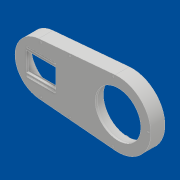
# Autodesk Inventor part: 101-bottom
Saved by Autodesk Inventor 2018 (Build 220112000, 112)
## iProperties
Created: 2019-11-07
Part Number: 101-bottom
Material: Generic
Document SubType Name: Modeling
Designer: Bunny320
Density: 1 g/cm^3
Appearance: Default
Author: Bunny320
Autodesk Inventor part; units mm, degrees
ref_plane "YZ Plane" through (0, 0, 0) normal (1, 0, 0) x (0, 1, 0)
ref_plane "XZ Plane" through (0, 0, 0) normal (0, 1, 0) x (-1, 0, 0)
ref_plane "XY Plane" through (0, 0, 0) normal (0, 0, 1) x (1, 0, 0)
sketch "Sketch2" plane through (0, 0, 0) normal (0, 1, 0) x (-1, 0, 0)
  circle A0 centre (0, 0) radius 45
  circle A1 centre (-141.8, 0) radius 57.5
  line L0 (3.9669, -44.8248) -> (-136.7312, -57.2762)
  line L1 (3.9669, 44.8248) -> (-136.7312, 57.2762)
  dimension "d5" = 141.8
  dimension "d6" = 90
  dimension "d7" = 115
  constraints: 4 end point, 4 point on circle, 4 tangent, 2 centre point, 1 coincident, 1 horizontal alignment
  measures "d5" distance of A1.centre point (0, 0)
  measures "d6" diameter of A0
  measures "d7" diameter of A1
extrude "Extrusion2" add sketch "Sketch2" along normal blind 4
sketch "Sketch5" plane through (0, 4, 0) normal (0, 1, 0) x (1, 0, 0)
  arc A0 (136.7312, -57.2762) -> (136.7312, 57.2762) centre (141.8, 0) ccw projected
  circle A1 centre (141.8, 0) radius 45
  circle A2 centre (141.8, 0) radius 48
  point P0 (0, 0)
  dimension "d17" = 90
  dimension "d18" = 96
  constraints: 2 centre point, 2 coincident
  measures "d17" diameter of A1
  measures "d18" diameter of A2
extrude "Extrusion5" add sketch "Sketch5" along normal blind 14
sketch "Sketch6" plane through (141.8, 4, 0) normal (0, 1, 0) x (1, 0, 0)
  arc A0 (-5.0688, -57.2762) -> (-5.0688, 57.2762) centre (0, 0) ccw projected
  circle A1 centre (0, 0) radius 42
  point P0 (-141.8, 0)
  dimension "d21" = 84
  constraints: 1 centre point, 1 coincident
  measures "d21" diameter of A1
extrude "Extrusion6" cut sketch "Sketch6" against normal through all
sketch "Sketch14" plane through (0, 0, 0) normal (0, 1, 0) x (-1, 0, 0)
  arc A0 (3.9669, -44.8248) -> (3.9669, 44.8248) centre (0, 0) ccw projected
  arc A1 (4.2313, -47.8131) -> (4.2313, 47.8131) centre (0, 0) ccw
  arc A2 (-136.7312, 57.2762) -> (-136.7312, -57.2762) centre (-141.8, 0) ccw projected
  arc A3 (-136.4668, 60.2645) -> (-136.4668, -60.2645) centre (-141.8, 0) ccw
  line L0 (4.2313, -47.8131) -> (-136.4668, -60.2645)
  line L1 (-136.4668, 60.2645) -> (4.2313, 47.8131)
  line L2 (-136.8194, -56.28) -> (3.8787, -43.8287)
  arc A4 (3.8787, -43.8287) -> (3.8787, 43.8287) centre (0, 0) ccw
  line L3 (3.8787, 43.8287) -> (-136.8194, 56.28)
  arc A5 (-136.8194, 56.28) -> (-136.8194, -56.28) centre (-141.8, 0) ccw
  dimension "d53" = 3
  dimension "d54" = 3
  dimension "d55" = 4
  constraints: 8 end point, 8 point on circle, 4 centre point, 4 tangent, 2 coincident, 3 other
  measures "d53" radial gap between concentric circles of A0 A1
  measures "d54" radial gap between concentric circles of A2 A3
  measures "d55" distance between parallel lines of L2 L0
extrude "Extrusion11" add sketch "Sketch14" along normal blind 26
sketch "Sketch21" plane through (0, 4, 0) normal (0, 1, 0) x (1, 0, 0)
  line L0 (-25, 23) -> (25, 23) construction
  line L1 (-25, 21.3) -> (25, 21.3)
  line L2 (25, 24.7) -> (-25, 24.7)
  arc A0 (-25, 24.7) -> (-25, 21.3) centre (-25, 23) ccw
  arc A1 (25, 21.3) -> (25, 24.7) centre (25, 23) ccw
  point P0 (0, 0)
  point P1 (0, 23)
  dimension "d113" = 3.4
  dimension "d116" = 50
  dimension "d117" = 23
  constraints: 8 end point, 4 point on circle, 4 tangent, 2 centre point, 1 horizontal, 1 midpoint, 1 parallel, 1 vertical alignment
  measures "d113" distance between parallel lines of L2 L1
  measures "d116" distance of L0.start L0.end
  measures "d117" distance from line of point (0, 0) L0
extrude "Extrusion15" cut sketch "Sketch21" against normal through all
sketch "Sketch22" plane through (0, 4, 0) normal (0, 1, 0) x (1, 0, 0)
  line L0 (-27, 29) -> (27, 29)
  line L1 (27, 29) -> (27, 26)
  line L2 (27, 26) -> (-27, 26)
  line L3 (-27, 26) -> (-27, 29)
  line L4 (-27, 29) -> (27, 26) construction
  line L5 (27, 29) -> (-27, 26) construction
  line L6 (-27, 20) -> (27, 20)
  line L7 (27, 20) -> (27, 17)
  line L8 (27, 17) -> (-27, 17)
  line L9 (-27, 17) -> (-27, 20)
  line L10 (-27, 20) -> (27, 17) construction
  line L11 (27, 20) -> (-27, 17) construction
  point P0 (0, 0)
  point P1 (0, 27.5)
  point P2 (0, 18.5)
  point P3 (0, 27.5)
  point P4 (0, 18.5)
  dimension "d118" = 6
  dimension "d119" = 3
  dimension "d120" = 3
  dimension "d121" = 26
  dimension "d122" = 54
  constraints: 24 end point, 6 midpoint, 4 parallel, 2 horizontal, 2 perpendicular, 2 vertical alignment, 1 point on line
  measures "d118" distance between parallel lines of L6 L2
  measures "d119" distance of L0.end L1.end
  measures "d120" distance of L6.end L7.end
  measures "d121" distance from line of point (0, 0) L2
  measures "d122" distance of L0.start L0.end
extrude "Extrusion16" add sketch "Sketch22" along normal blind 3
fillet "Fillet1" radius 2 4 edges at (0, 4, -29) (0, 4, -17) (0, 7, -17) (0, 7, -29)
mirror "Mirror2" about plane through (0, 0, 0) normal (0, 0, 1) of "Extrusion15", "Extrusion16", "Fillet1"
sketch "Sketch24" plane through (0, 4, 0) normal (0, 1, 0) x (1, 0, 0)
  line L0 (-27, -17.75) -> (27, -17.75)
  line L1 (27, -17.75) -> (27, 17.75)
  line L2 (27, 17.75) -> (-27, 17.75)
  line L3 (-27, 17.75) -> (-27, -17.75)
  line L4 (-27, -17.75) -> (27, 17.75) construction
  line L5 (27, -17.75) -> (-27, 17.75) construction
  point P0 (0, 0)
  dimension "d126" = 35.5
  dimension "d129" = 54
  constraints: 12 end point, 2 midpoint, 2 parallel, 1 horizontal, 1 perpendicular
  measures "d126" distance of L0.end L1.end
  measures "d129" distance of L1.end L2.end
extrude "Extrusion17" cut sketch "Sketch24" against normal through all
sketch "Sketch16" plane through (-3.8787, 4, 43.8287) normal (0.0882, 0, -0.9961) x (-0.9961, 0, -0.0882)
  line L0 (0, 0) -> (-141.248, 0) projected
  line L1 (0, 0) -> (-8, 0)
  line L2 (-8, 0) -> (-8, 22)
  line L3 (-8, 22) -> (0, 22)
  line L4 (0, 22) -> (0, 0)
  line L5 (-141.248, 22) -> (0, 22) projected
  line L6 (-53, 0) -> (-61, 0)
  line L7 (-61, 0) -> (-61, 22)
  line L8 (-61, 22) -> (-53, 22)
  line L9 (-53, 22) -> (-53, 0)
  point P0 (0, -4)
  dimension "d75" = 8
  dimension "d78" = 8
  dimension "d79" = 45
  constraints: 16 end point, 4 parallel, 2 horizontal, 2 perpendicular, 2 point on line, 1 collinear
  measures "d75" distance of L2.end L3.end
  measures "d78" distance between parallel lines of L7 L9
  measures "d79" distance between parallel lines of L9 L2
extrude "Extrusion12" add sketch "Sketch16" along normal blind 4 contours L0 L2 L3 L4 | L0 L7 L5 L9
sketch "Sketch17" plane through (0, 26, 0) normal (0, 1, 0) x (1, 0, 0)
  line L0 (-3.5261, -39.8443) -> (4.4428, -40.5495) projected
  line L1 (4.4428, -40.5495) -> (-5.0486, -46.5832)
  line L2 (-5.0486, -46.5832) -> (-3.356, -38.7638)
  line L3 (-3.356, -38.7638) -> (2.7501, -48.369)
  line L4 (48.915, -48.5008) -> (49.2676, -44.5164) projected
  line L5 (49.2676, -44.5164) -> (55.414, -53.9351)
  line L6 (49.2676, -44.5164) -> (57.2364, -45.2216) projected
  line L7 (57.2364, -45.2216) -> (48.5623, -52.4858)
  point P0 (0, 0)
  point P1 (-0.3029, -43.5664)
  point P2 (52.8994, -48.8537)
  constraints: 10 end point, 2 midpoint, 1 perpendicular, 1 point on line
hole "Hole4" at (-0.3029, 26, 43.5664) at (52.8994, 26, 48.8537) direction (0, -1, 0) diameter 2.459 end through all thread size "M3x0.5" class "6H" standard "ISO Metric profile"
mirror "Mirror1" about plane through (0, 0, 0) normal (0, 0, 1) of "Extrusion12", "Hole4"
sketch "Sketch18" plane through (0, 4, 0) normal (0, 1, 0) x (1, 0, 0)
  line L0 (193.8, -4) -> (201.8, -4)
  line L1 (201.8, -4) -> (201.8, 4)
  line L2 (201.8, 4) -> (193.8, 4)
  line L3 (193.8, 4) -> (193.8, -4)
  line L4 (193.8, -4) -> (201.8, 4) construction
  line L5 (201.8, -4) -> (193.8, 4) construction
  arc A0 (136.8194, -56.28) -> (136.8194, 56.28) centre (141.8, 0) ccw projected
  line L6 (136.8194, -56.28) -> (128.8505, -55.5748)
  line L7 (128.8505, -55.5748) -> (129.2031, -51.5904)
  line L8 (129.2031, -51.5904) -> (137.172, -52.2956)
  line L9 (137.172, -52.2956) -> (136.8194, -56.28)
  line L10 (136.8194, 56.28) -> (128.8505, 55.5748)
  line L11 (128.8505, 55.5748) -> (129.2031, 51.5904)
  line L12 (129.2031, 51.5904) -> (137.172, 52.2956)
  line L13 (137.172, 52.2956) -> (136.8194, 56.28)
  line L14 (56.8838, 49.206) -> (136.8194, 56.28) projected
  point P0 (0, 0)
  point P1 (197.8, 0)
  dimension "d87" = 8
  dimension "d89" = 4
  dimension "d90" = 4
  dimension "d92" = 8
  dimension "d93" = 8
  dimension "d112" = 56
  constraints: 28 end point, 6 parallel, 4 perpendicular, 2 midpoint, 1 collinear, 1 horizontal, 1 horizontal alignment, 1 tangent
  measures "d87" distance between parallel lines of L0 L2
  measures "d89" distance of L10.end L11.end
  measures "d90" distance of L6.end L7.end
  measures "d92" distance of L7.end L8.end
  measures "d93" distance of L11.end L12.end
  measures "d112" distance of A0.centre point (197.8, 0)
extrude "Extrusion13" add sketch "Sketch18" along normal up to surface (22 mm away)
sketch "Sketch19" plane through (0, 26, 0) normal (0, 1, 0) x (1, 0, 0)
  line L0 (128.8505, -55.5748) -> (56.8838, -49.206) projected
  line L1 (56.8838, 49.206) -> (128.8505, 55.5748) projected
  line L2 (129.2031, 51.5904) -> (128.8505, 55.5748) projected
  line L3 (128.8505, -55.5748) -> (129.2031, -51.5904) projected
  circle A0 centre (141.8, 0) radius 48 projected
  point P0 (0, 0)
  point P1 (132.835, 55.9274)
  point P2 (132.835, -55.9274)
  point P3 (197.8, 0)
  dimension "d99" = 56
  dimension "d131" = 4
  dimension "d132" = 4
  constraints: 2 point on line, 1 horizontal alignment
  measures "d99" distance of A0.centre point (197.8, 0)
  measures "d131" distance from line of L3 point (132.835, -55.927)
  measures "d132" distance from line of L2 point (132.835, 55.927)
hole "Hole5" at (132.835, 26, -55.9274) at (132.835, 26, 55.9274) at (197.8, 26, 0) direction (0, -1, 0) diameter 2.459 end through all thread size "M3x0.5" class "6H" standard "ISO Metric profile"
fillet "Fillet2" radius 2 28 edges at (-3.8787, 15, -43.8287) (-3.5261, 15, -39.8443) (4.4428, 15, -40.5495) (4.0902, 15, -44.5339) (48.915, 15, -48.5008) (49.2676, 15, -44.5164) (57.2364, 15, -45.2216) (56.8838, 15, -49.206) (137.172, 15, -52.2956) (129.2031, 15, -51.5904) (128.8505, 15, -55.5748) (136.8194, 15, -56.28) (193.8, 15, -4) (198.1582, 15, -4) (193.8, 15, 4) (198.1582, 15, 4) (136.8194, 15, 56.28) (129.2031, 15, 51.5904) (137.172, 15, 52.2956) (128.8505, 15, 55.5748) (56.8838, 15, 49.206) (57.2364, 15, 45.2216) (48.915, 15, 48.5008) (49.2676, 15, 44.5164) (-3.5261, 15, 39.8443) (-3.8787, 15, 43.8287) (4.0902, 15, 44.5339) (4.4428, 15, 40.5495)
equation "\"d54\" = d53"
equation "\"d120\" = d119"
equation "\"d121\" = d117 + 0.5 * d118"
equation "\"d78\" = d75"
equation "\"d89\" = d90"
equation "\"d93\" = d92"
equation "\"d132\" = d131"
body "Solid2"
